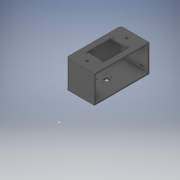
# Autodesk Inventor part: maincontrolpackage_third_eye_not_blind
Saved by Autodesk Inventor 2019 (Build 230136000, 136)
## iProperties
Created: 2019-02-05
Part Number: maincontrolpackage_third_eye_not_blind
Material: Generic
Document SubType Name: Modeling
Designer: ybharatu
Density: 1 g/cm^3
Appearance: Silicon Nitride - Polished
Author: ybharatu
Autodesk Inventor part; units mm, degrees
ref_plane "YZ Plane" through (0, 0, 0) normal (1, 0, 0) x (0, 1, 0)
ref_plane "XZ Plane" through (0, 0, 0) normal (0, 1, 0) x (-1, 0, 0)
ref_plane "XY Plane" through (0, 0, 0) normal (0, 0, 1) x (1, 0, 0)
sketch "Sketch1" plane through (0, 0, 0) normal (0, 1, 0) x (-1, 0, 0)
  line L0 (122.8458, -138.2757) -> (56.882, -138.2757)
  line L1 (56.882, -138.2757) -> (56.882, -265.2757)
  line L2 (56.882, -265.2757) -> (122.8458, -265.2757)
  line L3 (122.8458, -265.2757) -> (122.8458, -138.2757)
  line L4 (110.1458, -173.9373) -> (69.582, -173.9373)
  line L5 (69.582, -173.9373) -> (69.582, -229.6141)
  line L6 (69.582, -229.6141) -> (110.1458, -229.6141)
  line L7 (110.1458, -229.6141) -> (110.1458, -173.9373)
  point P0 (0, 0)
  dimension "d1" = 127
  dimension "d4" = 55.6768
  dimension "d5" = 40.5638
  dimension "d6" = 12.7
  dimension "d7" = 35.6616
  dimension "d8" = 12.7
  constraints: 16 end point, 4 parallel, 2 horizontal, 2 perpendicular
  measures "d1" distance of L2.end L0.start
  measures "d4" distance of L6.end L4.start
  measures "d5" distance of L5.end L6.end
  measures "d6" distance between parallel lines of L3 L7
  measures "d7" distance between parallel lines of L0 L4
  measures "d8" distance between parallel lines of L5 L1
extrude "Extrusion1" add sketch "Sketch1" along normal blind 63.5 contours L3 L2 L1 L0 | L7 L6 L5 L4
shell "Shell1" thickness 2.54 removed faces 1 at (-56.882, 21.1667, -180.609)
sketch "Sketch3" plane through (0, 63.5, 0) normal (0, 1, 0) x (1, 0, 0)
  line L0 (-110.1458, 174.0389) -> (-69.582, 174.0389)
  line L1 (-69.582, 174.0389) -> (-69.582, 229.7157)
  line L2 (-69.582, 229.7157) -> (-110.1458, 229.7157)
  line L3 (-110.1458, 229.7157) -> (-110.1458, 174.0389)
  line L4 (-122.8458, 265.2757) -> (-122.8458, 138.2757) projected
  line L5 (-56.882, 265.2757) -> (-122.8458, 265.2757) projected
  point P0 (0, 0)
  dimension "d14" = 55.6768
  dimension "d15" = 40.5638
  dimension "d16" = 12.7
  dimension "d17" = 35.56
  constraints: 8 end point, 2 parallel, 1 horizontal, 1 perpendicular
  measures "d14" distance of L2.end L0.start
  measures "d15" distance of L0.start L0.end
  measures "d16" distance between parallel lines of L4 L3
  measures "d17" distance between parallel lines of L5 L2
extrude "Extrusion2" cut sketch "Sketch3" against normal blind 12.7
sketch "Sketch4" plane through (0, 63.5, 0) normal (0, 1, 0) x (1, 0, 0)
  circle A0 centre (-91.0958, 156.2589) radius 2.4257
  line L0 (-69.582, 174.0389) -> (-110.1458, 174.0389) projected
  line L1 (-122.8458, 265.2757) -> (-122.8458, 138.2757) projected
  line L2 (-122.8458, 138.2757) -> (-56.882, 138.2757) projected
  line L3 (-69.582, 229.7157) -> (-69.582, 174.0389) projected
  line L4 (-69.582, 174.0389) -> (-110.1458, 174.0389) projected
  line L5 (-110.1458, 174.0389) -> (-110.1458, 229.7157) projected
  line L6 (-110.1458, 229.7157) -> (-69.582, 229.7157) projected
  line L7 (-122.8458, 138.2757) -> (-56.882, 138.2757) projected
  line L8 (-56.882, 138.2757) -> (-56.882, 265.2757) projected
  line L9 (-56.882, 265.2757) -> (-122.8458, 265.2757) projected
  line L10 (-122.8458, 265.2757) -> (-122.8458, 138.2757) projected
  circle A1 centre (-91.0958, 247.4957) radius 2.4257
  point P0 (0, 0)
  dimension "d20" = 4.8514
  dimension "d21" = 17.78
  dimension "d22" = 31.75
  dimension "d23" = 4.8514
  dimension "d24" = 17.78
  dimension "d25" = 31.75
  constraints: 2 centre point
  measures "d20" diameter of A0
  measures "d21" distance from line of L0 A0.centre
  measures "d22" distance from line of L1 A0.centre
  measures "d23" diameter of A1
  measures "d24" distance from line of A1.centre L6
  measures "d25" distance from line of L1 A1.centre
hole "Hole1" at (-91.0958, 63.5, -156.2589) at (-91.0958, 63.5, -247.4957) direction (0, -1, 0) diameter 4.8514 depth 12.7 tip angle 118
sketch "Sketch5" plane through (0, 0, 0) normal (0, -1, 0) x (1, 0, 0)
  line L0 (-122.8458, -265.2757) -> (-122.8458, -138.2757) projected
  line L1 (-122.8458, -138.2757) -> (-56.882, -138.2757) projected
  line L2 (-122.8458, -265.2757) -> (-122.8458, -138.2757) projected
  line L3 (-56.882, -265.2757) -> (-122.8458, -265.2757) projected
  line L4 (-56.882, -138.2757) -> (-56.882, -265.2757) projected
  line L5 (-96.1758, -206.0937) -> (-87.5398, -206.0937)
  line L6 (-87.5398, -206.0937) -> (-87.5398, -197.4577)
  line L7 (-87.5398, -197.4577) -> (-96.1758, -197.4577)
  line L8 (-96.1758, -197.4577) -> (-96.1758, -206.0937)
  circle A0 centre (-91.8578, -191.8951) radius 1.0414
  circle A1 centre (-91.8578, -212.4032) radius 1.0826
  point P0 (0, 0)
  dimension "d33" = 8.636
  dimension "d34" = 8.636
  dimension "d35" = 26.67
  dimension "d36" = 59.182
  dimension "d64" = 2.0828
  dimension "d65" = 5.5626
  dimension "d83" = 127
  dimension "d84" = 8.636
  constraints: 8 end point, 2 centre point, 2 parallel, 1 horizontal, 1 perpendicular
  measures "d33" distance of L7.end L5.start
  measures "d34" distance of L5.start L5.end
  measures "d35" distance between parallel lines of L0 L8
  measures "d36" distance between parallel lines of L5 L3
  measures "d64" diameter of A0
  measures "d65" distance from line of A0.centre L7
  measures "d83" distance of L1.end L3.start
  measures "d84" distance of L5.end L6.end
extrude "Extrusion3" cut sketch "Sketch5" against normal blind 12.7 contours L8 L7 L6 L5
sketch "Sketch6" plane through (-122.8458, 0, -265.2757) normal (-1, 0, 0) x (0, 0, 1)
  circle A0 centre (63.5, 50.8) radius 3.556
  line L0 (127, 0) -> (127, 63.5) projected
  line L1 (0, 63.5) -> (127, 63.5) projected
  line L2 (116.7244, 19.05) -> (97.1664, 19.05)
  line L3 (97.1664, 19.05) -> (97.1664, 6.35)
  line L4 (97.1664, 6.35) -> (116.7244, 6.35)
  line L5 (116.7244, 6.35) -> (116.7244, 19.05)
  line L6 (0, 0) -> (127, 0) projected
  point P0 (265.2757, 0)
  dimension "d39" = 7.112
  dimension "d40" = 63.5
  dimension "d41" = 12.7
  dimension "d49" = 12.7
  dimension "d50" = 19.558
  dimension "d51" = 6.35
  constraints: 8 end point, 2 parallel, 1 centre point, 1 horizontal, 1 perpendicular
  measures "d39" diameter of A0
  measures "d40" distance from line of L0 A0.centre
  measures "d41" distance from line of L1 A0.centre
  measures "d49" distance of L4.end L2.start
  measures "d50" distance of L2.start L2.end
  measures "d51" distance between parallel lines of L6 L4
hole "Hole2" at (-122.8458, 50.8, -201.7757) direction (1, 0, 0) diameter 7.112 depth 12.7 tip angle 118
extrude "Extrusion4" cut sketch "Sketch6" against normal blind 12.7 contours L5 L4 L3 L2
fillet "Fillet1" radius 6.35 2 edges at (-122.8458, 31.75, -265.2757) (-122.8458, 31.75, -138.2757)
sketch "Sketch8" plane through (0, 63.5, 0) normal (0, 1, 0) x (1, 0, 0)
  point P0 (0, 0)
sketch "Sketch9" plane through (0, 63.5, 0) normal (0, 1, 0) x (1, 0, 0)
  point P0 (0, 0)
sketch "Sketch10" plane through (0, 63.5, 0) normal (0, 1, 0) x (1, 0, 0)
  line L0 (-110.1458, 229.7157) -> (-69.582, 229.7157) projected
  line L1 (-110.1458, 174.0389) -> (-110.1458, 229.7157) projected
  line L2 (-69.582, 229.7157) -> (-69.582, 174.0389) projected
  line L3 (-69.582, 174.0389) -> (-110.1458, 174.0389) projected
  point P0 (0, 0)
  point P1 (-107.301, 232.5605)
  point P2 (-72.4268, 232.5605)
  point P3 (-107.301, 171.1941)
  point P4 (-72.4268, 171.1941)
  dimension "d66" = 2.8448
  dimension "d67" = 2.8448
  dimension "d68" = 2.8448
  dimension "d69" = 2.8448
  dimension "d70" = 2.8448
  dimension "d71" = 2.8448
  dimension "d72" = 2.8448
  dimension "d73" = 2.8448
  measures "d66" distance from line of L0 point (-107.301, 232.56)
  measures "d67" distance from line of L1 point (-107.301, 232.56)
  measures "d68" distance from line of point (-72.427, 232.56) L2
  measures "d69" distance from line of L0 point (-72.427, 232.56)
  measures "d70" distance from line of L3 point (-107.301, 171.194)
  measures "d71" distance from line of L1 point (-107.301, 171.194)
  measures "d72" distance from line of L3 point (-72.427, 171.194)
  measures "d73" distance from line of L2 point (-72.427, 171.194)
hole "Hole4" at (-72.4268, 63.5, -232.5605) at (-107.301, 63.5, -171.1941) at (-72.4268, 63.5, -171.1941) at (-107.301, 63.5, -232.5605) direction (0, -1, 0) diameter 2.6416 depth 12.7 tip angle 118
sketch "Sketch11" plane through (0, 0, 0) normal (0, -1, 0) x (1, 0, 0)
  line L0 (-106.285, -214.7297) -> (-82.155, -214.7297)
  line L1 (-82.155, -214.7297) -> (-82.155, -189.3297)
  line L2 (-82.155, -189.3297) -> (-106.285, -189.3297)
  line L3 (-106.285, -189.3297) -> (-106.285, -214.7297)
  line L4 (-96.1758, -206.0937) -> (-96.1758, -197.4577) projected
  line L5 (-96.1758, -197.4577) -> (-87.5398, -197.4577) projected
  line L6 (-87.5398, -206.0937) -> (-96.1758, -206.0937) projected
  point P0 (0, 0)
  point P1 (-104.2022, -191.4125)
  point P2 (-104.2022, -212.6469)
  point P3 (-91.6292, -212.6469)
  point P4 (-91.6292, -191.4125)
  dimension "d81" = 24.13
  dimension "d82" = 25.4
  dimension "d85" = 14.0208
  dimension "d87" = 16.764
  dimension "d88" = 2.0828
  dimension "d89" = 2.0828
  dimension "d90" = 2.0828
  dimension "d91" = 2.0828
  dimension "d92" = 2.0828
  dimension "d93" = 2.0828
  dimension "d95" = 12.573
  dimension "d96" = 12.573
  constraints: 8 end point, 2 parallel, 1 horizontal, 1 perpendicular
  measures "d81" distance of L1.end L2.end
  measures "d82" distance of L2.end L0.start
  measures "d85" distance between parallel lines of L4 L1
  measures "d87" distance between parallel lines of L2 L6
  measures "d88" distance from line of L2 point (-104.202, -191.412)
  measures "d89" distance from line of L3 point (-104.202, -191.412)
  measures "d90" distance from line of L3 point (-104.202, -212.647)
  measures "d91" distance from line of L0 point (-104.202, -212.647)
  measures "d92" distance from line of L0 point (-91.629, -212.647)
  measures "d93" distance from line of L2 point (-91.629, -191.412)
  measures "d95" distance of point (-91.629, -191.412) point (-104.202, -191.412)
  measures "d96" distance of point (-104.202, -212.647) point (-91.629, -212.647)
hole "Hole5" at (-104.2022, 0, -212.6469) at (-104.2022, 0, -191.4125) at (-91.6292, 0, -191.4125) at (-91.6292, 0, -212.6469) direction (0, 1, 0) diameter 2.286 depth 12.7 tip angle 118
sketch "Sketch14" plane through (-56.882, 0, -265.2757) normal (0, 0, -1) x (-1, 0, 0)
  line L0 (17.78, 13.2334) -> (10.16, 13.2334)
  line L1 (10.16, 13.2334) -> (10.16, 10.16)
  line L2 (10.16, 10.16) -> (17.78, 10.16)
  line L3 (17.78, 10.16) -> (17.78, 13.2334)
  line L4 (0, 2.54) -> (63.4238, 2.54) projected
  line L5 (0, 0) -> (0, 63.5) projected
  point P0 (-56.882, 0)
  dimension "d114" = 7.62
  dimension "d115" = 3.0734
  dimension "d116" = 7.62
  dimension "d117" = 10.16
  constraints: 8 end point, 2 parallel, 1 horizontal, 1 perpendicular
  measures "d114" distance between parallel lines of L4 L2
  measures "d115" distance between parallel lines of L2 L0
  measures "d116" distance of L0.start L0.end
  measures "d117" distance from line of L0.end L5
extrude "Extrusion6" cut sketch "Sketch14" against normal blind 12.7
equation "\"d7\" = -0.5 * d4 + 0.5 * d1"
equation "\"d8\" = d6"
equation "\"d36\" = 0.5 * d83 - 0.5 * d84"
body "Solid1"
